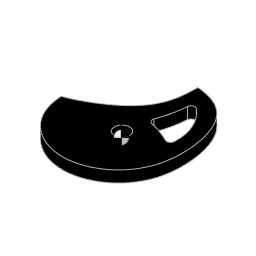
Weapon-5in (Autodesk Fusion 360 design; units mm, degrees)
Autodesk Fusion 360 part; units mm, degrees
sketch "Sketch1" plane through (0, 0, 0) normal (0, 0, 1) x (1, 0, 0)
  circle A0 centre (0, 0) radius 127 construction
  circle A1 centre (0, 0) radius 101.6 construction
  circle A2 centre (0, 0) radius 12.7
  line L0 (0, -141.6667) -> (0, 141.6667) construction
  line L1 (-170, 0) -> (170, 0) construction
  spline S0 degree 5 poles (0, 127) (0, 125.4788) (-0.0177, 122.257) (-0.0972, 116.8859) (-0.3989, 108.7197) (-1.5971, 97.2581) (-4.2051, 85.0941) (-8.738, 72.808) (-15.4433, 60.9012) (-24.1564, 49.7136) (-34.4456, 39.4692) (-45.7073, 30.3015) (-57.2694, 22.2807) (-68.4816, 15.4341) (-78.8164, 9.7638) (-87.9482, 5.261) (-94.1442, 2.5834) (-98.1309, 1.0913) (-100.4929, 0.3256) (-101.6, 0) knots 0 0 0 0 0 0 0.066667 0.133333 0.2 0.266667 0.333333 0.4 0.466667 0.533333 0.6 0.666667 0.733333 0.8 0.866667 0.933333 1 1 1 1 1 1
  line L2 (-87.4333, 4.1667) -> (-115.7667, -4.1667)
  line L3 (0, 143.6469) -> (0, 110.3531)
  spline S1 degree 5 poles (0, 127) (0.2871, 127) (1.8405, 126.9) (7.108, 126.4503) (18.9813, 124.8162) (36.9466, 119.0461) (53.3534, 107.7515) (66.5714, 90.7405) (75.8896, 69.1059) (81.4017, 44.6566) (83.305, 19.3723) (81.729, -4.9389) (75.6549, -27.5607) (64.5061, -47.9243) (48.6255, -65.1605) (28.7704, -78.33) (6.0804, -86.434) (-18.2709, -88.3871) (-42.9865, -83.3334) (-65.9914, -71.4303) (-85.0746, -53.2436) (-95.5299, -34.3083) (-99.9658, -17.9529) (-101.3221, -6.1365) (-101.6, 0) knots 0 0 0 0 0 0 0.05 0.1 0.15 0.2 0.25 0.3 0.35 0.4 0.45 0.5 0.55 0.6 0.65 0.7 0.75 0.8 0.85 0.9 0.95 1 1 1 1 1 1
  line L4 (-4.9396, 127) -> (4.9396, 127)
  line L5 (4.3366, 138.047) -> (78.9967, 91.5752)
  line L6 (42.8356, -79.6866) -> (-42.8356, -92.1286)
  line L7 (-99.2089, -52.7983) -> (-103.9911, 52.7983)
  line L8 (87.2673, 46.4826) -> (75.2803, -46.4826)
  circle A3 centre (25.4043, 90.2761) radius 6.35
  circle A4 centre (14.9592, 42.4227) radius 6.35
  circle A5 centre (52.3674, 29.0626) radius 6.35
  arc A6 (58.7073, 28.7043) -> (29.4195, 95.1955) centre (-21.1653, 33.2182) ccw
  arc A7 (49.5252, 23.3842) -> (13.5611, 36.2285) centre (-21.2545, -118.0273) ccw
  arc A8 (9.0222, 44.6754) -> (19.0686, 90.7021) centre (-140.5708, 101.4375) ccw
  point P0 (-8.3333, 75)
  point P1 (-66.6667, 16.6667)
  point P2 (41.6667, 114.8111)
  point P3 (81.2738, 0)
  point P4 (0, -85.9076)
  dimension "d3" = 25.4
  dimension "d13" = 203.2
  dimension "d14" = 12.7
  dimension "d15" = 12.7
  dimension "d16" = 12.7
  dimension "d17" = 80
  dimension "d18" = 160
  constraint coincident A0.centre A1.centre
  constraint concentric A0 A1
  constraint vertical L0
  constraint horizontal L1
  constraint coincident A0 S0.start
  constraint coincident L0 S0.start
  constraint coincident A1 S0.end
  constraint coincident L1 S0.end
  constraint midpoint S0.end L2
  constraint midpoint S0.start L3
  constraint coincident L0 L3.end
  constraint coincident L1 P3
  constraint midpoint S0.start L4
  constraint midpoint P2 L5
  constraint midpoint P4 L6
  constraint midpoint S0.end L7
  constraint midpoint P3 L8
  constraint coincident A1 L6.end
  constraint coincident A0.centre L0
  constraint coincident A0.centre L1
  constraint coincident L0 P4
  constraint coincident A5 A6.start
  constraint coincident A3 A6.end
  constraint tangent A3 A6
  constraint tangent A5 A6
  constraint tangent A4 A7
  constraint coincident A5 A7.start
  constraint coincident A4 A7.end
  constraint tangent A4 A8
  constraint coincident A3 A8.end
  constraint coincident A4 A8.start
  constraint tangent A3 A8
  constraint tangent A5 A7
  measures "d3" diameter of A2
  measures "d13" diameter of A1
  measures "d14" diameter of A3
  measures "d15" diameter of A4
  measures "d16" diameter of A5
  measures "d17" radius of A6
  measures "d18" radius of A8
extrude "Extrude1" add sketch "Sketch1" along normal blind 19.05
